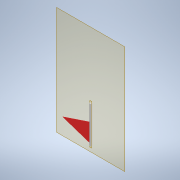
# Autodesk Inventor part: flag holder
Saved by Autodesk Inventor 2020.3 (Build 243373000, 373)
## iProperties
Created: 2021-03-04
Part Number: flag holder
Material: Generic
Document SubType Name: Modeling
Designer: con_c_000
Density: 1 g/cm^3
Appearance: Default
Author: con_c_000
Autodesk Inventor part; units mm, degrees
ref_plane "YZ Plane" through (0, 0, 0) normal (1, 0, 0) x (0, 1, 0)
ref_plane "XZ Plane" through (0, 0, 0) normal (0, 1, 0) x (-1, 0, 0)
ref_plane "XY Plane" through (0, 0, 0) normal (0, 0, 1) x (1, 0, 0)
ref_plane "Work Plane1" through (0, 0, 0) normal (0, 0, 1) x (1, 0, 0)
sketch "Sketch1" plane through (0, 0, 0) normal (0, 0, 1) x (1, 0, 0)
  line L0 (0, -789.9925) -> (25.4, -789.9925)
  line L1 (25.4, -789.9925) -> (25.4, -180.3925)
  line L2 (25.4, -180.3925) -> (0, -180.3925)
  line L3 (0, -180.3925) -> (0, -789.9925)
  point P0 (0, 0)
  dimension "d0" = 25.4
  dimension "d1" = 609.6
  constraints: 8 end point, 2 parallel, 1 horizontal, 1 perpendicular
  measures "d0" distance of L2.end L1.end
  measures "d1" distance of L1.end L0.end
extrude "Extrusion1" add sketch "Sketch1" along normal blind 25.4
ref_plane "Work Plane2" through (0, 0, 12.7) normal (0, 0, 1) x (1, 0, 0)
sketch "Sketch3" plane through (0, 0, 12.7) normal (0, 0, 1) x (1, 0, 0)
  line L0 (0, -180.3925) -> (0, -789.9925) projected
  line L1 (0, -761.3575) -> (0, -456.5575)
  line L2 (0, -456.5575) -> (-457.2, -608.9575)
  line L3 (-457.2, -608.9575) -> (0, -761.3575)
  point P0 (0, 0)
  dimension "d8" = 304.8
  dimension "d9" = 457.2
  constraints: 6 end point, 2 point on line
  measures "d8" distance of L1.start L1.end
  measures "d9" horizontal distance of L2.end L1.end
extrude "Extrusion2" add sketch "Sketch3" along normal mid plane 2.54
body "Solid1"
